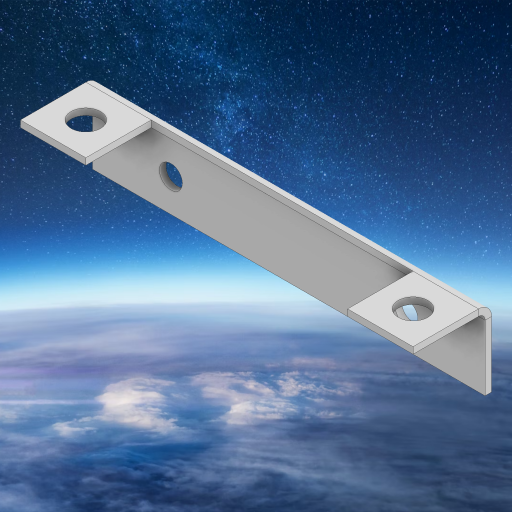
# Autodesk Inventor part: fan_fix_plate_connect
Saved by Autodesk Inventor 2023 (Build 270158000, 158)
## iProperties
Created: 2023-10-03
Part Number: fan_fix_plate_connect
Material: Generic
Document SubType Name: Sheet Metal
Designer: 310611102
Density: 1 g/cm^3
Sheet Metal Rule: Default_mm
Appearance: Default
Author: 310611102
Autodesk Inventor part; units mm, degrees
ref_plane "YZ Plane" through (0, 0, 0) normal (1, 0, 0) x (0, 1, 0)
ref_plane "XZ Plane" through (0, 0, 0) normal (0, 1, 0) x (-1, 0, 0)
ref_plane "XY Plane" through (0, 0, 0) normal (0, 0, 1) x (1, 0, 0)
sketch "Sketch1" plane through (0, 0, 0) normal (0, 0, 1) x (1, 0, 0)
  line L0 (-30, 5) -> (30, 5)
  line L1 (30, 5) -> (30, -5)
  line L2 (30, -5) -> (-30, -5)
  line L3 (-30, -5) -> (-30, 5)
  line L4 (-30, 5) -> (30, -5) construction
  line L5 (30, 5) -> (-30, -5) construction
  circle A0 centre (-18, 0) radius 1.75
  line L6 (0, 0) -> (0, -5.5046) construction
  circle A1 centre (18, 0) radius 1.75
  dimension "d0" = 60
  dimension "d1" = 10
  dimension "d2" = 3.5
  dimension "d3" = 36
  dimension "d4" = 5
  measures "d0" distance of L0.start L0.end
  measures "d1" distance of L0.end L1.end
  measures "d2" diameter of A0
  measures "d3" distance of A1.centre A0.centre
  measures "d4" distance from line of L2 A0.centre
extrude "Plate1" add sketch "Sketch1" along normal blind 1
sketch "Sketch2" plane through (-30, 6, 2) normal (0, 1, 0) x (-1, 0, 0)
  line L0 (-60, 0) -> (0, 0)
  line L1 (0, 0) -> (0, 10)
  line L2 (0, 10) -> (-60, 10)
  line L3 (-60, 10) -> (-60, 0)
  constraints: 6 end point, 1 horizontal, 1 perpendicular, 1 vertical
edge flange "Flange1" height 12 angle 90 thickness 1 bend radius 1 thickness toward (0, 1, 0) relief tear relief width 1 relief depth 0.5 edges at (0, 5, 1) wall of the first edge with corners at (30, 6, 2) (-30, 6, 2) (-30, 6, 12) (30, 6, 12)
bend "Bend1"
corner "Corner1"
sketch "Sketch3" plane through (-30, 6, 12) normal (0, -1, 0) x (1, 0, 0)
  circle A0 centre (55, -5) radius 2.25
  circle A1 centre (5, -5) radius 2.25
  line L0 (30, -12) -> (30, 5.1941) construction
  line L1 (60, -11) -> (0, -11) construction
  dimension "d20" = 4.5
  dimension "d21" = 4.5
  dimension "d22" = 50
  dimension "d23" = 6
  constraints: 2 centre point, 2 end point, 1 symmetric about line, 1 vertical
  measures "d20" diameter of A0
  measures "d21" diameter of A1
  measures "d22" distance of A1.centre A0.centre
  measures "d23" distance from line of L1 A0.centre
extrude "Cut1" cut sketch "Sketch3" against normal blind 1
sketch "Sketch4" plane through (-30, 7, 12) normal (0, 1, 0) x (1, 0, 0)
  line L0 (60, 0) -> (0, 0) projected
  line L1 (50, 10) -> (10, 10)
  line L2 (10, 10) -> (10, 0)
  line L3 (10, 0) -> (50, 0)
  line L4 (50, 0) -> (50, 10)
  line L5 (50, 10) -> (10, 0) construction
  line L6 (10, 10) -> (50, 0) construction
  line L7 (60, 10) -> (0, 10) projected
  point P0 (30, 12)
  point P1 (30, 5)
  dimension "d26" = 40
  constraints: 12 end point, 2 midpoint, 2 parallel, 1 collinear, 1 horizontal, 1 perpendicular, 1 point on line, 1 vertical alignment
  measures "d26" distance between parallel lines of L4 L2
extrude "Cut2" cut sketch "Sketch4" against normal blind 1
equation "\"d20\" = d21"
equation "\"d24\" = 厚度"
equation "\"d27\" = 厚度"
equation "\"d9\" = 厚度"
equation "\"d10\" = 折彎離隙寬度"
equation "\"d11\" = 折彎離隙深度"
equation "\"d12\" = 最小剩餘"
equation "\"d13\" = 轉移半徑"
equation "\"d16\" = 折彎半徑"
equation "\"d17\" = 轉角離隙大小"
equation "\"d18\" = 間隙大小"
equation "\"d19\" = Jacobi半徑大小"
equation "\"折彎半徑\" = 厚度"
equation "\"折彎離隙寬度\" = 厚度"
equation "\"折彎離隙深度\" = 0.5 * 厚度"
equation "\"轉角離隙大小\" = 4 * 厚度"
equation "\"最小剩餘\" = 2 * 厚度"
equation "\"轉移半徑\" = 折彎半徑"
equation "\"Jacobi半徑大小\" = 折彎半徑"
equation "\"間隙大小\" = 厚度"
equation "\"厚度\" = 1"
body "Solid1"
